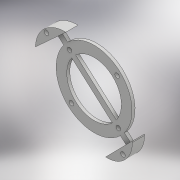
# Autodesk Inventor part: SoporteAnilloRGB
Saved by Autodesk Inventor 2017 (Build 210142000, 142)
## iProperties
Created: 2018-06-26
Part Number: SoporteAnilloRGB
Material: Generic
Document SubType Name: Modeling
Designer: Carolina Lema
Density: 1 g/cm^3
Appearance: Default
Author: Carolina Lema
Autodesk Inventor part; units mm, degrees
ref_plane "YZ Plane" through (0, 0, 0) normal (1, 0, 0) x (0, 1, 0)
ref_plane "XZ Plane" through (0, 0, 0) normal (0, 1, 0) x (-1, 0, 0)
ref_plane "XY Plane" through (0, 0, 0) normal (0, 0, 1) x (1, 0, 0)
sketch "Sketch1" plane through (0, 0, 0) normal (0, 1, 0) x (-1, 0, 0)
  line L0 (27.5685, -23.1529) -> (7.584, -4.7581)
  line L1 (27.5685, -23.1529) -> (7.584, -4.7581)
  spline S0 degree 3 poles (7.584, -4.7581) (9.0341, -4.7222) (10.4847, -4.8305) (13.3346, -5.3449) (14.7272, -5.7489) (18.2487, -7.2033) (20.2523, -8.489) (23.6504, -11.7447) (25.0047, -13.6664) (26.9871, -18.1293) (27.5054, -20.6082) (27.5685, -23.1529) knots -2.481768 -2.481768 -2.481768 -2.481768 -2.126999 -2.126999 -1.773298 -1.773298 -1.19466 -1.19466 -0.620796 -0.620796 0 0 0 0
  circle A0 centre (20.3262, -11.4054) radius 1.5
  line L2 (-36.2673, -45.7716) -> (-36.2673, -44.9248)
  spline S1 degree 3 poles (-19.9806, -62.8419) (-22.0219, -62.8419) (-24.0395, -62.4476) (-27.9058, -60.8796) (-29.6966, -59.6913) (-32.7933, -56.6261) (-34.0383, -54.7586) (-35.8128, -50.509) (-36.2673, -48.1535) (-36.2673, -45.7716) knots -2.639853 -2.639853 -2.639853 -2.639853 -2.025479 -2.025479 -1.383917 -1.383917 -0.714589 -0.714589 0 0 0 0
  line L3 (-18.6392, -62.8419) -> (-19.9806, -62.8419)
  line L4 (-18.6392, -62.8419) -> (-36.2673, -44.9248)
  circle A1 centre (-30.091, -55.5905) radius 1.5
  point P0 (0, 0)
  point P1 (4.2097, 0)
  constraints: 10 end point, 2 centre point, 4 other
extrude "Extrusion1" add sketch "Sketch1" along normal blind 8
sketch "Sketch2" plane through (0, 8, 0) normal (0, 1, 0) x (1, 0, 0)
  circle A0 centre (-20.3262, 11.4054) radius 1.5 projected
  circle A1 centre (30.091, 55.5905) radius 1.5 projected
  line L0 (-19.1981, 12.3941) -> (-17.7266, 11.0396)
  line L1 (-7.584, 4.7581) -> (-27.5685, 23.1529) projected
  line L2 (-17.7266, 11.0396) -> (-20.6696, 13.7485)
  line L3 (-20.6696, 13.7485) -> (27.4533, 56.3244)
  line L4 (27.4533, 56.3244) -> (30.0896, 53.3162)
  line L5 (-17.7266, 11.0396) -> (30.0896, 53.3162)
  point P0 (0, 0)
  dimension "d2" = 2
  dimension "d3" = 4
  dimension "d4" = 4
  constraints: 10 end point, 1 parallel, 1 point on line, 2 other
  measures "d2" distance of L0.start L0.end
  measures "d3" distance of L0.end L2.end
  measures "d4" distance of L3.end L4.end
extrude "Extrusion2" add sketch "Sketch2" against normal blind 2 contours L2 A0 | A0 L2 L3 L1 L5 L0 | L1 L3 L4 L5 picked at (-19.3013, 12.4925)
sketch "Sketch3" plane through (0, 8, 0) normal (0, 1, 0) x (1, 0, 0)
  circle A0 centre (5.0339, 33.8258) radius 25
  circle A1 centre (5.0339, 33.8258) radius 18
  circle A2 centre (-11.1078, 19.6239) radius 1.5
  circle A3 centre (-9.8663, 49.3253) radius 1.5
  circle A4 centre (20.2206, 18.607) radius 1.5
  circle A5 centre (21.1064, 48.106) radius 1.5
  point P0 (0, 0)
  dimension "d9" = 3
  dimension "d10" = 3
  dimension "d11" = 3
  dimension "d12" = 3
  constraints: 6 centre point, 1 coincident
  measures "d9" diameter of A2
  measures "d10" diameter of A3
  measures "d11" diameter of A4
  measures "d12" diameter of A5
extrude "Extrusion3" add sketch "Sketch3" against normal blind 2
sketch "Sketch4" plane through (0, 8, 0) normal (0, 1, 0) x (1, 0, 0)
  circle A0 centre (5.0339, 33.8258) radius 25
  circle A1 centre (5.0339, 33.8258) radius 18
  circle A2 centre (-11.1078, 19.6239) radius 1.5
  circle A3 centre (-9.8663, 49.3253) radius 1.5
  circle A4 centre (20.2206, 18.607) radius 1.5
  circle A5 centre (21.1064, 48.106) radius 1.5
  point P0 (0, 0)
  point P1 (0, 0)
  dimension "d15" = 3
  dimension "d16" = 3
  dimension "d17" = 3
  dimension "d18" = 3
  constraints: 6 centre point, 1 coincident
  measures "d15" diameter of A2
  measures "d16" diameter of A3
  measures "d17" diameter of A4
  measures "d18" diameter of A5
extrude "Extrusion4" cut sketch "Sketch4" against normal blind 2 contours A2 | A5
body "Solid1"
